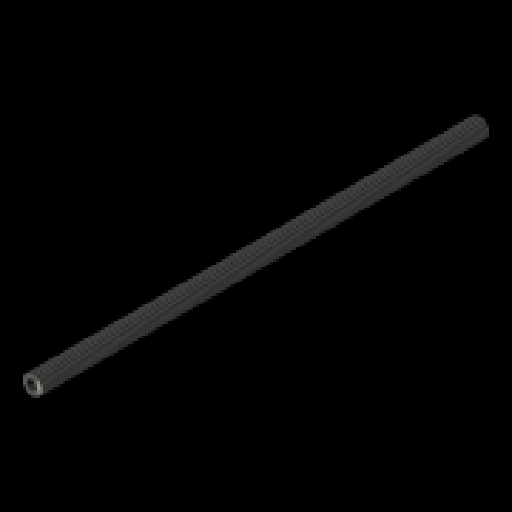
# Autodesk Inventor part: RodMK3
Saved by Autodesk Inventor 2025 (Build 290162000, 162)
## iProperties
Created: 2024-11-11
Part Number: RodMK3
Material: Stainless Steel
Document SubType Name: Modeling
Designer: Trevor
Density: 8 g/cm^3
Appearance: Semi-Polished
Author: Trevor
Autodesk Inventor part; units mm, degrees
ref_plane "YZ Plane" through (0, 0, 0) normal (1, 0, 0) x (0, 1, 0)
ref_plane "XZ Plane" through (0, 0, 0) normal (0, 1, 0) x (-1, 0, 0)
ref_plane "XY Plane" through (0, 0, 0) normal (0, 0, 1) x (1, 0, 0)
sketch "Sketch1" plane through (0, 0, 0) normal (0, 0, 1) x (1, 0, 0)
  circle A0 centre (0, 0) radius 2.5 projected
  circle A1 centre (0, 0) radius 4.9
  point P0 (0, 0)
  dimension "d0" = 9.8
  constraints: 1 centre point, 1 coincident
  measures "d0" diameter of A1
ref_plane "Work Plane1" through (-33.85, -16.15, 180) normal (0, 0, -1) x (0, 1, 0)
extrude "Extrusion1" add sketch "Sketch1" along normal blind 227.564
thread "Thread1" size "M10x1.5" class "6g" standard "ANSI Metric M Profile" full length
body "Solid1"
